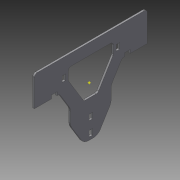
# Autodesk Inventor part: Top Plate 27100914
Saved by Autodesk Inventor 2015 (Build 190159000, 159)
## iProperties
Created: 2011-09-22
Part Number: Top Plate 27100914
Document SubType Name: Modeling
Designer: user
Density: 1 g/cm^3
Material: Generic
Appearance: Default
Author: user
Autodesk Inventor part; units mm, degrees
ref_plane "YZ Plane" through (0, 0, 0) normal (1, 0, 0) x (0, 1, 0)
ref_plane "XZ Plane" through (0, 0, 0) normal (0, 1, 0) x (-1, 0, 0)
ref_plane "XY Plane" through (0, 0, 0) normal (0, 0, 1) x (1, 0, 0)
sketch "Sketch2" plane through (0, 0, 0) normal (0, 1, 0) x (-1, 0, 0)
  line L0 (70, -18) -> (60, -18)
  line L1 (60, -18) -> (60, -12)
  line L2 (70, -12) -> (70, -18)
  line L3 (-70, -18.0006) -> (-60, -18.0006)
  line L4 (-60, -18.0006) -> (-60, -12.0003)
  line L5 (-70, -12.0003) -> (-70, -18.0006)
  line L6 (3, 70) -> (-3, 70)
  line L7 (-3, 70) -> (-3, 80)
  line L8 (-3, 80) -> (3, 80)
  line L9 (3, 80) -> (3, 70)
  line L10 (3, 45) -> (-3, 45)
  line L11 (-3, 45) -> (-3, 55)
  line L12 (-3, 55) -> (3, 55)
  line L13 (3, 55) -> (3, 45)
  line L14 (95, -65) -> (-95, -65)
  line L15 (-12.5, 85) -> (12.5, 85)
  line L16 (12.5, 85) -> (35.9015, 46.7742)
  line L17 (-100, -12.0003) -> (-70, -12.0003)
  line L18 (-55.4919, -12.0003) -> (-60, -12.0003)
  line L19 (55.4917, -12) -> (60, -12)
  line L20 (70, -12) -> (100, -12)
  line L21 (-100, -60) -> (-100, -12.0003)
  line L22 (100, -60) -> (100, -12)
  line L23 (35, -45) -> (-35, -45)
  line L24 (-40, -40) -> (-40, -26.409)
  line L25 (-39.2644, -23.7983) -> (-13.9141, 17.6106)
  line L26 (-9.6497, 20) -> (9.6497, 20)
  line L27 (40, -40) -> (40, -26.409)
  line L28 (39.2644, -23.7983) -> (13.9141, 17.6106)
  arc A0 (-40, -40) -> (-35, -45) centre (-35, -40) ccw
  arc A1 (-39.2644, -23.7983) -> (-40, -26.409) centre (-35, -26.409) ccw
  arc A2 (-9.6497, 20) -> (-13.9141, 17.6106) centre (-9.6497, 15) ccw
  arc A3 (13.9141, 17.6106) -> (9.6497, 20) centre (9.6497, 15) ccw
  arc A4 (40, -26.409) -> (39.2644, -23.7983) centre (35, -26.409) ccw
  arc A5 (35, -45) -> (40, -40) centre (35, -40) ccw
  line L29 (55.4917, -12) -> (35.9015, 20)
  line L30 (35.9015, 20) -> (35.9015, 46.7742)
  line L31 (-55.4919, -12.0003) -> (-35.9015, 20)
  line L32 (-35.9015, 20) -> (-35.9015, 46.7742)
  line L33 (-35.9015, 46.7742) -> (-12.5, 85)
  line L34 (0, -65) -> (0, 85) construction
  arc A6 (95, -65) -> (100, -60) centre (95, -60) ccw
  arc A7 (-100, -60) -> (-95, -65) centre (-95, -60) ccw
  point P0 (100, -65)
  point P1 (-100, -65)
  point P2 (0, 0)
  point P3 (0, 80)
  point P4 (0, 45)
  point P5 (0, 55)
  point P6 (0, 0)
  point P7 (0, 0)
  point P8 (-70, -15.4178)
  point P9 (75.3708, -12)
  point P10 (0, 0)
  point P11 (-40, -45)
  point P12 (40, -45)
  point P13 (-40, -25)
  point P14 (-12.4513, 20)
  point P15 (12.4513, 20)
  point P16 (40, -25)
  point P17 (0, 20)
  point P18 (0, -45)
  dimension "d65" = 200
  dimension "d115" = 10
  dimension "d116" = 6
  dimension "d118" = 10
  dimension "d119" = 6
  dimension "d120" = 15
  dimension "d147" = 65
  dimension "d173" = 25
  dimension "d187" = 100
  dimension "d191" = 30
  dimension "d192" = 30
  dimension "d194" = 6.0003
  dimension "d195" = 6
  dimension "d196" = 10
  dimension "d197" = 10
  dimension "d198" = 52.9997
  dimension "d199" = 53
  dimension "d204" = 150
  dimension "d213" = 20
  dimension "d214" = 20
  dimension "d218" = 65
  dimension "d219" = 40
  dimension "d220" = 5
  dimension "d233" = 148.525
  dimension "d235" = 5
  dimension "d236" = 20
  dimension "d249" = 5
  constraints: 70 end point, 18 point on line, 16 point on circle, 16 tangent, 12 parallel, 9 perpendicular, 8 centre point, 8 midpoint, 6 equal radius, 5 coincident, 5 horizontal, 5 vertical alignment, 4 horizontal alignment, 2 collinear, 2 vertical, 5 other
  measures "d65" distance of point (100, -65) point (-100, -65)
  measures "d115" distance of L6.end L7.end
  measures "d116" distance of L7.end L8.end
  measures "d118" distance of L12.end L10.start
  measures "d119" distance of L10.start L10.end
  measures "d120" distance between parallel lines of L6 L12
  measures "d147" distance from line of point (0, 0) L14
  measures "d173" distance of L15.start L15.end
  measures "d187" horizontal distance of point (0, 0) point (-100, -65)
  measures "d191" distance of L17.start L5.start
  measures "d192" distance of L2.start L20.end
  measures "d194" distance of L5.start L3.start
  measures "d195" distance of L2.start L0.start
  measures "d196" distance of L3.start L3.end
  measures "d197" distance of L0.start L0.end
  measures "d198" distance of point (-100, -65) L17.start
  measures "d199" distance of point (100, -65) L20.end
  measures "d204" distance between parallel lines of L14 L15
  measures "d213" distance between parallel lines of L14 L23
  measures "d214" distance of point (-40, -45) point (-40, -25)
  measures "d218" distance between parallel lines of L23 L26
  measures "d219" distance from line of point (0, 0) L24
  measures "d220" radius of A0
  measures "d233" angle of L24 L25
  measures "d235" distance between parallel lines of L15 L8
  measures "d236" distance between parallel lines of L28 L29
  measures "d249" radius of A6
extrude "Extrusion11" add sketch "Sketch2" along normal blind 3
sketch "Sketch4" plane through (0, 3, 0) normal (0, 1, 0) x (1, 0, 0)
  line L0 (-51, 38) -> (-45, 38)
  line L1 (-45, 38) -> (-45, 28)
  line L2 (-45, 28) -> (-51, 28)
  line L3 (-51, 28) -> (-51, 38)
  line L4 (95, 65) -> (-95, 65) projected
  line L5 (-40, 40) -> (-40, 26.409) projected
  line L6 (45, 38) -> (51, 38)
  line L7 (51, 38) -> (51, 28)
  line L8 (51, 28) -> (45, 28)
  line L9 (45, 28) -> (45, 38)
  line L10 (40, 40) -> (40, 26.409) projected
  point P0 (0, 0)
  point P1 (100, 65)
  point P2 (-100, 65)
  dimension "d237" = 6
  dimension "d238" = 27
  dimension "d239" = 10
  dimension "d240" = 5
  dimension "d241" = 6
  dimension "d242" = 10
  dimension "d243" = 5
  dimension "d244" = 27
  constraints: 16 end point, 4 parallel, 2 horizontal, 2 perpendicular
  measures "d237" distance of L0.start L0.end
  measures "d238" distance between parallel lines of L4 L0
  measures "d239" distance of L2.end L0.start
  measures "d240" distance between parallel lines of L5 L1
  measures "d241" distance of L7.end L8.end
  measures "d242" distance of L6.end L7.end
  measures "d243" distance between parallel lines of L10 L9
  measures "d244" distance between parallel lines of L4 L6
extrude "Extrusion13" cut sketch "Sketch4" against normal through all
fillet "Fillet1" radius 15 6 edges at (12.5, 1.5, 85) (-12.5, 1.5, 85) (-35.9015, 1.5, 46.7742) (35.9015, 1.5, 46.7742) (35.9015, 1.5, 20) (-35.9015, 1.5, 20)
fillet "Fillet2" radius 5 2 edges at (55.4919, 1.5, -12.0003) (-55.4917, 1.5, -12)
body "Solid11"
